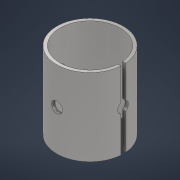
# Autodesk Inventor part: Test_Blade_Holder
Saved by Autodesk Inventor 2022 (Build 260153000, 153)
## iProperties
Created: 2024-05-09
Part Number: Test_Blade_Holder
Material: Generic
Document SubType Name: Modeling
Designer: jo_ki
Density: 1 g/cm^3
Appearance: Stainless - Brushed
Author: jo_ki
Autodesk Inventor part; units mm, degrees
note: some values were not read from the file. Chosen so that the rebuilt part matches the saved one: pattern direction of "Circular Pattern1".
ref_plane "YZ Plane" through (0, 0, 0) normal (1, 0, 0) x (0, 1, 0)
ref_plane "XZ Plane" through (0, 0, 0) normal (0, 1, 0) x (-1, 0, 0)
sketch "Sketch2" plane through (0, 0, 0) normal (0, 1, 0) x (-1, 0, 0)
  circle A0 centre (0, 0) radius 14
  circle A1 centre (0, 0) radius 12.7
  line L0 (0, -19.6) -> (0, 19.6) projected
  line L1 (-12.6606, -1) -> (-13.9642, -1)
  line L2 (-13.9642, 1) -> (-12.6606, 1)
  line L3 (19.6, 0) -> (-19.6, 0) projected
  dimension "d3" = 25.4
  dimension "d4" = 28
  dimension "d19" = 2
  dimension "d20" = 1.3
  constraints: 4 end point, 4 point on circle, 2 centre point, 2 coincident, 1 horizontal, 1 parallel, 1 other
  measures "d3" diameter of A1
  measures "d4" diameter of A0
  measures "d19" distance between parallel lines of L1 L2
  measures "d20" radial gap between concentric circles of A1 A0
extrude "Extrusion1" add sketch "Sketch2" along normal mid plane 32.5 contours L3 A1 L0 A0 | A0 L0 A1 L3 | L0 A1 L2 A0 | A0 L1 A1 L0
ref_plane "Work Plane1" through (0, 0, 14) normal (0, 0, 1) x (1, 0, 0)
sketch "Sketch3" plane through (0, 0, 14) normal (0, 0, 1) x (1, 0, 0)
  line L0 (-14, -16.25) -> (13.9642, -16.25) projected
  line L1 (0, -22.75) -> (0, 22.75) projected
  point P0 (0, 0)
  point P1 (0, 0.75)
  dimension "d8" = 17
  constraints: 1 point on line
  measures "d8" distance from line of L0 point (0, 0.75)
hole "Hole1" at (0, 0.75, 14) direction (0, 0, -1) diameter 4.5 depth 10 clearance for "Socket Head Cap Screw DIN EN ISO 4762" size "M4" standard "DIN"
pattern_circular "Circular Pattern1" count 3 over 180 about axis through (0, -10, 0) along (0, 1, 0) of "Hole1" both ways yes
body "Solid1"
